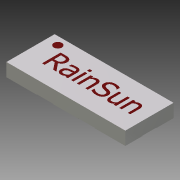
# Autodesk Inventor part: MD1506
Saved by Autodesk Inventor 2015 SP1 (Build 190203100, 203)
## iProperties
Created: 2015-01-30
Part Number: MD1506
Material: Типовые
Document SubType Name: Modeling
Designer: Danil
Density: 1 g/cm^3
Appearance: Полированная поверхность — серебряная
Author: Danil
Autodesk Inventor part; units mm, degrees
ref_plane "YZ Plane" through (0, 0, 0) normal (1, 0, 0) x (0, 1, 0)
ref_plane "XZ Plane" through (0, 0, 0) normal (0, 1, 0) x (-1, 0, 0)
sketch "Эскиз1" plane through (0, 0, 0) normal (0, 0, 1) x (1, 0, 0)
  line L0 (7.4, -3) -> (-7.4, -3)
  line L1 (-7.4, -3) -> (-7.4, 3)
  line L2 (-7.4, 3) -> (7.4, 3)
  line L3 (7.4, 3) -> (7.4, -3)
  line L4 (7.4, -3) -> (-7.4, 3) construction
  line L5 (-7.4, -3) -> (7.4, 3) construction
  line L6 (-7.4, 3) -> (-3.6, 3)
  line L7 (-3.6, 3) -> (-3.6, 0.9)
  line L8 (-3.6, 0.9) -> (-7.4, 0.9)
  line L9 (-7.4, 0.9) -> (-7.4, 3)
  line L10 (-7.4, -3) -> (-3.6, -3)
  line L11 (-3.6, -3) -> (-3.6, -0.9)
  line L12 (-3.6, -0.9) -> (-7.4, -0.9)
  line L13 (-7.4, -0.9) -> (-7.4, -3)
  line L14 (7.4, 3) -> (3.6, 3)
  line L15 (3.6, 3) -> (3.6, 0.9)
  line L16 (3.6, 0.9) -> (7.4, 0.9)
  line L17 (7.4, 0.9) -> (7.4, 3)
  line L18 (7.4, -3) -> (3.6, -3)
  line L19 (3.6, -3) -> (3.6, -0.9)
  line L20 (3.6, -0.9) -> (7.4, -0.9)
  line L21 (7.4, -0.9) -> (7.4, -3)
  line L22 (-1.6, 3) -> (1.6, 3)
  line L23 (1.6, 3) -> (1.6, 0.9)
  line L24 (1.6, 0.9) -> (-1.6, 0.9)
  line L25 (-1.6, 0.9) -> (-1.6, 3)
  line L26 (-1.6, -3) -> (1.6, -3)
  line L27 (1.6, -3) -> (1.6, -0.9)
  line L28 (1.6, -0.9) -> (-1.6, -0.9)
  line L29 (-1.6, -0.9) -> (-1.6, -3)
  circle A0 centre (-5.6325, 1.95) radius 0.6107
  point P0 (0, 0)
  dimension "d2" = 14.8
  dimension "d3" = 6
  dimension "d4" = 3.8
  dimension "d5" = 2.1
  dimension "d6" = 3.8
  dimension "d7" = 2.1
  dimension "d8" = 3.8
  dimension "d9" = 2.1
  dimension "d10" = 3.8
  dimension "d11" = 2.1
  dimension "d12" = 3.2
  dimension "d13" = 2.1
  dimension "d14" = 3.2
  dimension "d15" = 2.1
  constraints: 60 end point, 14 parallel, 7 horizontal, 7 perpendicular, 3 point on line, 2 midpoint, 1 centre point
  measures "d2" distance of L1.end L2.end
  measures "d3" distance of L0.end L1.end
  measures "d4" distance of L7.end L8.end
  measures "d5" distance of L6.end L7.end
  measures "d6" distance of L12.end L11.end
  measures "d7" distance of L11.end L10.end
  measures "d8" distance of L16.end L15.end
  measures "d9" distance of L15.end L14.end
  measures "d10" distance of L19.end L20.end
  measures "d11" distance of L18.end L19.end
  measures "d12" distance of L23.end L24.end
  measures "d13" distance of L22.end L23.end
  measures "d14" distance of L28.end L27.end
  measures "d15" distance of L27.end L26.end
extrude "Выдавливание1" add sketch "Эскиз1" along normal blind 1.6 contours L0 L19 L20 L3 | L0 L27 L28 L29 L11 L12 L1 L8 L7 L2 L25 L24 L23 L15 L16 L3 L20 L19 | L0 L29 L28 L27 | L16 L15 L2 L3 | L0 L1 L12 L11 | L23 L24 L25 L2 | L1 L2 L7 L8 | A0
extrude "Выдавливание2" add sketch "Эскиз1" against normal blind 0.05 contours L0 L19 L20 L3 | L0 L29 L28 L27 | L16 L15 L2 L3 | L0 L1 L12 L11 | L23 L24 L25 L2 | L1 L2 L7 L8 | A0
ref_plane "РабПлоскость1" through (0, 0, 1.6) normal (0, 0, 1) x (1, 0, 0)
sketch "Эскиз2" plane through (0, 0, 1.6) normal (0, 0, 1) x (1, 0, 0)
  circle A0 centre (-6.0059, 2.0006) radius 0.5
  line L0 (-5.2655, 1.417) -> (6.3838, 1.417) construction
  line L1 (6.3838, 1.417) -> (6.3838, -1.2479) construction
  line L2 (6.3838, -1.2479) -> (-5.2655, -1.2479) construction
  line L3 (-5.2655, -1.2479) -> (-5.2655, 1.417) construction
  line L4 (-3.2525, -0.924) -> (-3.6495, -0.924)
  line L5 (-3.6495, -0.924) -> (-4.3764, -0.0089)
  line L6 (-4.3764, -0.0089) -> (-4.7268, -0.0089)
  line L7 (-4.7268, -0.0089) -> (-4.7268, -0.924)
  line L8 (-4.7268, -0.924) -> (-5.0325, -0.924)
  line L9 (-5.0325, -0.924) -> (-5.0325, 1.376)
  line L10 (-5.0325, 1.376) -> (-4.4398, 1.376)
  spline S0 degree 2 poles (-4.4398, 1.376) (-4.2422, 1.376) (-3.9757, 1.3331) (-3.8545, 1.2548) knots 0 0 0 1 2 2 2
  spline S1 degree 2 poles (-3.8545, 1.2548) (-3.7334, 1.1766) (-3.5936, 0.9324) (-3.5936, 0.7516) knots 0 0 0 1 2 2 2
  spline S2 degree 2 poles (-3.5936, 0.7516) (-3.5936, 0.5) (-3.8508, 0.1589) (-4.0707, 0.0769) knots 0 0 0 1 2 2 2
  line L11 (-4.0707, 0.0769) -> (-3.2525, -0.924)
  spline S3 degree 2 poles (-3.9123, 0.7274) (-3.9123, 0.828) (-3.9831, 0.9827) (-4.0577, 1.033) knots 0 0 0 1 2 2 2
  spline S4 degree 2 poles (-4.0577, 1.033) (-4.1229, 1.0759) (-4.2962, 1.1113) (-4.423, 1.1113) knots 0 0 0 1 2 2 2
  line L12 (-4.423, 1.1113) -> (-4.7268, 1.1113)
  line L13 (-4.7268, 1.1113) -> (-4.7268, 0.2465)
  line L14 (-4.7268, 0.2465) -> (-4.4584, 0.2465)
  spline S5 degree 2 poles (-4.4584, 0.2465) (-4.3261, 0.2465) (-4.1155, 0.2931) (-4.0428, 0.3658) knots 0 0 0 1 2 2 2
  spline S6 degree 2 poles (-4.0428, 0.3658) (-3.9757, 0.4291) (-3.9123, 0.6081) (-3.9123, 0.7274) knots 0 0 0 1 2 2 2
  spline S7 degree 2 poles (-2.1304, -0.7414) (-2.1659, -0.7674) (-2.2851, -0.8606) (-2.3411, -0.8886) knots 0 0 0 1 2 2 2
  spline S8 degree 2 poles (-2.3411, -0.8886) (-2.4175, -0.9296) (-2.561, -0.9725) (-2.6915, -0.9725) knots 0 0 0 1 2 2 2
  spline S9 degree 2 poles (-2.6915, -0.9725) (-2.7977, -0.9725) (-2.9897, -0.8923) (-3.0624, -0.8196) knots 0 0 0 1 2 2 2
  spline S10 degree 2 poles (-3.0624, -0.8196) (-3.1313, -0.7488) (-3.2152, -0.5401) (-3.2152, -0.4245) knots 0 0 0 1 2 2 2
  spline S11 degree 2 poles (-3.2152, -0.4245) (-3.2152, -0.2456) (-3.0642, 0.0079) (-2.9002, 0.0806) knots 0 0 0 1 2 2 2
  spline S12 degree 2 poles (-2.9002, 0.0806) (-2.7548, 0.1477) (-2.3597, 0.198) (-2.1304, 0.2111) knots 0 0 0 1 2 2 2
  line L15 (-2.1304, 0.2111) -> (-2.1304, 0.267)
  spline S13 degree 2 poles (-2.1304, 0.267) (-2.1304, 0.3676) (-2.1919, 0.4925) (-2.2479, 0.5279) knots 0 0 0 1 2 2 2
  spline S14 degree 2 poles (-2.2479, 0.5279) (-2.3038, 0.5633) (-2.4641, 0.5857) (-2.5498, 0.5857) knots 0 0 0 1 2 2 2
  spline S15 degree 2 poles (-2.5498, 0.5857) (-2.6505, 0.5857) (-2.9226, 0.5261) (-3.0586, 0.4683) knots 0 0 0 1 2 2 2
  line L16 (-3.0586, 0.4683) -> (-3.0754, 0.4683)
  line L17 (-3.0754, 0.4683) -> (-3.0754, 0.7646)
  spline S16 degree 2 poles (-3.0754, 0.7646) (-2.9953, 0.787) (-2.6952, 0.8429) (-2.5479, 0.8429) knots 0 0 0 1 2 2 2
  spline S17 degree 2 poles (-2.5479, 0.8429) (-2.369, 0.8429) (-2.1249, 0.787) (-2.0279, 0.7143) knots 0 0 0 1 2 2 2
  spline S18 degree 2 poles (-2.0279, 0.7143) (-1.9329, 0.6435) (-1.8397, 0.418) (-1.8397, 0.2558) knots 0 0 0 1 2 2 2
  line L18 (-1.8397, 0.2558) -> (-1.8397, -0.924)
  line L19 (-1.8397, -0.924) -> (-2.1304, -0.924)
  line L20 (-2.1304, -0.924) -> (-2.1304, -0.7414)
  line L21 (-2.1304, -0.4991) -> (-2.1304, -0.02)
  spline S19 degree 2 poles (-2.1304, -0.02) (-2.2348, -0.0294) (-2.5498, -0.061) (-2.6486, -0.0909) knots 0 0 0 1 2 2 2
  spline S20 degree 2 poles (-2.6486, -0.0909) (-2.7642, -0.1263) (-2.9151, -0.2735) (-2.9151, -0.404) knots 0 0 0 1 2 2 2
  spline S21 degree 2 poles (-2.9151, -0.404) (-2.9151, -0.5531) (-2.7474, -0.7041) (-2.5871, -0.7041) knots 0 0 0 1 2 2 2
  spline S22 degree 2 poles (-2.5871, -0.7041) (-2.451, -0.7041) (-2.2274, -0.5867) (-2.1304, -0.4991) knots 0 0 0 1 2 2 2
  line L22 (-1.1351, -0.924) -> (-1.4259, -0.924)
  line L23 (-1.4259, -0.924) -> (-1.4259, 0.8019)
  line L24 (-1.4259, 0.8019) -> (-1.1351, 0.8019)
  line L25 (-1.1351, 0.8019) -> (-1.1351, -0.924)
  line L26 (-1.1146, 1.089) -> (-1.4445, 1.089)
  line L27 (-1.4445, 1.089) -> (-1.4445, 1.3909)
  line L28 (-1.4445, 1.3909) -> (-1.1146, 1.3909)
  line L29 (-1.1146, 1.3909) -> (-1.1146, 1.089)
  line L30 (0.6467, -0.924) -> (0.3559, -0.924)
  line L31 (0.3559, -0.924) -> (0.3559, 0.0601)
  spline S23 degree 2 poles (0.3559, 0.0601) (0.3559, 0.1794) (0.3336, 0.3844) (0.3, 0.4459) knots 0 0 0 1 2 2 2
  spline S24 degree 2 poles (0.3, 0.4459) (0.2646, 0.5112) (0.1379, 0.5745) (0.0298, 0.5745) knots 0 0 0 1 2 2 2
  spline S25 degree 2 poles (0.0298, 0.5745) (-0.0783, 0.5745) (-0.3076, 0.459) (-0.4176, 0.3658) knots 0 0 0 1 2 2 2
  line L32 (-0.4176, 0.3658) -> (-0.4176, -0.924)
  line L33 (-0.4176, -0.924) -> (-0.7083, -0.924)
  line L34 (-0.7083, -0.924) -> (-0.7083, 0.8019)
  line L35 (-0.7083, 0.8019) -> (-0.4176, 0.8019)
  line L36 (-0.4176, 0.8019) -> (-0.4176, 0.6099)
  spline S26 degree 2 poles (-0.4176, 0.6099) (-0.2871, 0.7274) (-0.0355, 0.8504) (0.1062, 0.8504) knots 0 0 0 1 2 2 2
  spline S27 degree 2 poles (0.1062, 0.8504) (0.3597, 0.8504) (0.6467, 0.5149) (0.6467, 0.1962) knots 0 0 0 1 2 2 2
  line L37 (0.6467, 0.1962) -> (0.6467, -0.924)
  spline S28 degree 2 poles (1.7184, -0.965) (1.4687, -0.965) (1.1183, -0.8606) (0.9636, -0.7861) knots 0 0 0 1 2 2 2
  line L38 (0.9636, -0.7861) -> (0.9636, -0.4021)
  line L39 (0.9636, -0.4021) -> (0.9859, -0.4021)
  spline S29 degree 2 poles (0.9859, -0.4021) (1.1369, -0.5438) (1.519, -0.7003) (1.6961, -0.7003) knots 0 0 0 1 2 2 2
  spline S30 degree 2 poles (1.6961, -0.7003) (1.9495, -0.7003) (2.2086, -0.4897) (2.2086, -0.3164) knots 0 0 0 1 2 2 2
  spline S31 degree 2 poles (2.2086, -0.3164) (2.2086, -0.1785) (2.0726, -0.007) (1.9253, 0.0359) knots 0 0 0 1 2 2 2
  spline S32 degree 2 poles (1.9253, 0.0359) (1.8191, 0.0657) (1.642, 0.1067) (1.5097, 0.1402) knots 0 0 0 1 2 2 2
  spline S33 degree 2 poles (1.5097, 0.1402) (1.3904, 0.1719) (1.2021, 0.267) (1.1294, 0.3434) knots 0 0 0 1 2 2 2
  spline S34 degree 2 poles (1.1294, 0.3434) (1.0586, 0.4198) (0.9803, 0.6249) (0.9803, 0.7591) knots 0 0 0 1 2 2 2
  spline S35 degree 2 poles (0.9803, 0.7591) (0.9803, 1.0386) (1.4165, 1.417) (1.7538, 1.417) knots 0 0 0 1 2 2 2
  spline S36 degree 2 poles (1.7538, 1.417) (1.9477, 1.417) (2.2906, 1.3406) (2.4379, 1.2679) knots 0 0 0 1 2 2 2
  line L40 (2.4379, 1.2679) -> (2.4379, 0.9026)
  line L41 (2.4379, 0.9026) -> (2.4155, 0.9026)
  spline S37 degree 2 poles (2.4155, 0.9026) (2.3055, 1.0032) (1.9626, 1.1523) (1.7743, 1.1523) knots 0 0 0 1 2 2 2
  spline S38 degree 2 poles (1.7743, 1.1523) (1.5619, 1.1523) (1.2991, 0.9529) (1.2991, 0.7907) knots 0 0 0 1 2 2 2
  spline S39 degree 2 poles (1.2991, 0.7907) (1.2991, 0.6454) (1.4538, 0.472) (1.5991, 0.4329) knots 0 0 0 1 2 2 2
  spline S40 degree 2 poles (1.5991, 0.4329) (1.6961, 0.4068) (1.9775, 0.3397) (2.0707, 0.3117) knots 0 0 0 1 2 2 2
  spline S41 degree 2 poles (2.0707, 0.3117) (2.3074, 0.239) (2.5273, -0.0536) (2.5273, -0.2679) knots 0 0 0 1 2 2 2
  spline S42 degree 2 poles (2.5273, -0.2679) (2.5273, -0.404) (2.4174, -0.6649) (2.3186, -0.7563) knots 0 0 0 1 2 2 2
  spline S43 degree 2 poles (2.3186, -0.7563) (2.2086, -0.8569) (1.929, -0.965) (1.7184, -0.965) knots 0 0 0 1 2 2 2
  line L42 (4.1582, -0.924) -> (3.8675, -0.924)
  line L43 (3.8675, -0.924) -> (3.8675, -0.7339)
  spline S44 degree 2 poles (3.8675, -0.7339) (3.7333, -0.8513) (3.4928, -0.9725) (3.3437, -0.9725) knots 0 0 0 1 2 2 2
  spline S45 degree 2 poles (3.3437, -0.9725) (3.2319, -0.9725) (3.0324, -0.8979) (2.9598, -0.8178) knots 0 0 0 1 2 2 2
  spline S46 degree 2 poles (2.9598, -0.8178) (2.8852, -0.7376) (2.8032, -0.4935) (2.8032, -0.3183) knots 0 0 0 1 2 2 2
  line L44 (2.8032, -0.3183) -> (2.8032, 0.8019)
  line L45 (2.8032, 0.8019) -> (3.0939, 0.8019)
  line L46 (3.0939, 0.8019) -> (3.0939, -0.1822)
  spline S47 degree 2 poles (3.0939, -0.1822) (3.0939, -0.3201) (3.1145, -0.5009) (3.1499, -0.568) knots 0 0 0 1 2 2 2
  spline S48 degree 2 poles (3.1499, -0.568) (3.1853, -0.6351) (3.3064, -0.6966) (3.4201, -0.6966) knots 0 0 0 1 2 2 2
  spline S49 degree 2 poles (3.4201, -0.6966) (3.5264, -0.6966) (3.7668, -0.5755) (3.8675, -0.4879) knots 0 0 0 1 2 2 2
  line L47 (3.8675, -0.4879) -> (3.8675, 0.8019)
  line L48 (3.8675, 0.8019) -> (4.1582, 0.8019)
  line L49 (4.1582, 0.8019) -> (4.1582, -0.924)
  line L50 (5.9345, -0.924) -> (5.6437, -0.924)
  line L51 (5.6437, -0.924) -> (5.6437, 0.0601)
  spline S50 degree 2 poles (5.6437, 0.0601) (5.6437, 0.1794) (5.6213, 0.3844) (5.5878, 0.4459) knots 0 0 0 1 2 2 2
  spline S51 degree 2 poles (5.5878, 0.4459) (5.5524, 0.5112) (5.4256, 0.5745) (5.3175, 0.5745) knots 0 0 0 1 2 2 2
  spline S52 degree 2 poles (5.3175, 0.5745) (5.2094, 0.5745) (4.9802, 0.459) (4.8702, 0.3658) knots 0 0 0 1 2 2 2
  line L52 (4.8702, 0.3658) -> (4.8702, -0.924)
  line L53 (4.8702, -0.924) -> (4.5794, -0.924)
  line L54 (4.5794, -0.924) -> (4.5794, 0.8019)
  line L55 (4.5794, 0.8019) -> (4.8702, 0.8019)
  line L56 (4.8702, 0.8019) -> (4.8702, 0.6099)
  spline S53 degree 2 poles (4.8702, 0.6099) (5.0007, 0.7274) (5.2523, 0.8504) (5.3939, 0.8504) knots 0 0 0 1 2 2 2
  spline S54 degree 2 poles (5.3939, 0.8504) (5.6474, 0.8504) (5.9345, 0.5149) (5.9345, 0.1962) knots 0 0 0 1 2 2 2
  line L57 (5.9345, 0.1962) -> (5.9345, -0.924)
  dimension "d37" = 1
  constraints: 1 centre point, 2 other
  measures "d37" diameter of A0
extrude "Выдавливание3" add sketch "Эскиз2" along normal blind 0.01
